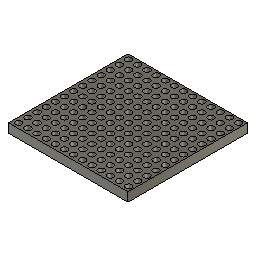
speakergrill_main__unit v1 (Autodesk Fusion 360 design; units mm, degrees)
Autodesk Fusion 360 part; units mm, degrees
sketch "Sketch1" plane through (0, 0, 0) normal (0, 0, 1) x (1, 0, 0)
  line L0 (-122.591, 65.2661) -> (-62.791, 65.2661)
  line L1 (-62.791, 65.2661) -> (-62.791, 5.4661)
  line L2 (-62.791, 5.4661) -> (-122.591, 5.4661)
  line L3 (-122.591, 5.4661) -> (-122.591, 65.2661)
  circle A0 centre (-120, 63) radius 1.5
  circle A1 centre (-115.4167, 63) radius 1.5
  circle A2 centre (-110.8333, 63) radius 1.5
  circle A3 centre (-106.25, 63) radius 1.5
  circle A4 centre (-101.6667, 63) radius 1.5
  circle A5 centre (-97.0833, 63) radius 1.5
  circle A6 centre (-92.5, 63) radius 1.5
  circle A7 centre (-87.9167, 63) radius 1.5
  circle A8 centre (-83.3333, 63) radius 1.5
  circle A9 centre (-78.75, 63) radius 1.5
  circle A10 centre (-74.1667, 63) radius 1.5
  circle A11 centre (-69.5833, 63) radius 1.5
  circle A12 centre (-65, 63) radius 1.5
  circle A13 centre (-120, 58.4167) radius 1.5
  circle A14 centre (-115.4167, 58.4167) radius 1.5
  circle A15 centre (-110.8333, 58.4167) radius 1.5
  circle A16 centre (-106.25, 58.4167) radius 1.5
  circle A17 centre (-101.6667, 58.4167) radius 1.5
  circle A18 centre (-97.0833, 58.4167) radius 1.5
  circle A19 centre (-92.5, 58.4167) radius 1.5
  circle A20 centre (-87.9167, 58.4167) radius 1.5
  circle A21 centre (-83.3333, 58.4167) radius 1.5
  circle A22 centre (-78.75, 58.4167) radius 1.5
  circle A23 centre (-74.1667, 58.4167) radius 1.5
  circle A24 centre (-69.5833, 58.4167) radius 1.5
  circle A25 centre (-65, 58.4167) radius 1.5
  circle A26 centre (-120, 53.8333) radius 1.5
  circle A27 centre (-115.4167, 53.8333) radius 1.5
  circle A28 centre (-110.8333, 53.8333) radius 1.5
  circle A29 centre (-106.25, 53.8333) radius 1.5
  circle A30 centre (-101.6667, 53.8333) radius 1.5
  circle A31 centre (-97.0833, 53.8333) radius 1.5
  circle A32 centre (-92.5, 53.8333) radius 1.5
  circle A33 centre (-87.9167, 53.8333) radius 1.5
  circle A34 centre (-83.3333, 53.8333) radius 1.5
  circle A35 centre (-78.75, 53.8333) radius 1.5
  circle A36 centre (-74.1667, 53.8333) radius 1.5
  circle A37 centre (-69.5833, 53.8333) radius 1.5
  circle A38 centre (-65, 53.8333) radius 1.5
  circle A39 centre (-120, 49.25) radius 1.5
  circle A40 centre (-115.4167, 49.25) radius 1.5
  circle A41 centre (-110.8333, 49.25) radius 1.5
  circle A42 centre (-106.25, 49.25) radius 1.5
  circle A43 centre (-101.6667, 49.25) radius 1.5
  circle A44 centre (-97.0833, 49.25) radius 1.5
  circle A45 centre (-92.5, 49.25) radius 1.5
  circle A46 centre (-87.9167, 49.25) radius 1.5
  circle A47 centre (-83.3333, 49.25) radius 1.5
  circle A48 centre (-78.75, 49.25) radius 1.5
  circle A49 centre (-74.1667, 49.25) radius 1.5
  circle A50 centre (-69.5833, 49.25) radius 1.5
  circle A51 centre (-65, 49.25) radius 1.5
  circle A52 centre (-120, 44.6667) radius 1.5
  circle A53 centre (-115.4167, 44.6667) radius 1.5
  circle A54 centre (-110.8333, 44.6667) radius 1.5
  circle A55 centre (-106.25, 44.6667) radius 1.5
  circle A56 centre (-101.6667, 44.6667) radius 1.5
  circle A57 centre (-97.0833, 44.6667) radius 1.5
  circle A58 centre (-92.5, 44.6667) radius 1.5
  circle A59 centre (-87.9167, 44.6667) radius 1.5
  circle A60 centre (-83.3333, 44.6667) radius 1.5
  circle A61 centre (-78.75, 44.6667) radius 1.5
  circle A62 centre (-74.1667, 44.6667) radius 1.5
  circle A63 centre (-69.5833, 44.6667) radius 1.5
  circle A64 centre (-65, 44.6667) radius 1.5
  circle A65 centre (-120, 40.0833) radius 1.5
  circle A66 centre (-115.4167, 40.0833) radius 1.5
  circle A67 centre (-110.8333, 40.0833) radius 1.5
  circle A68 centre (-106.25, 40.0833) radius 1.5
  circle A69 centre (-101.6667, 40.0833) radius 1.5
  circle A70 centre (-97.0833, 40.0833) radius 1.5
  circle A71 centre (-92.5, 40.0833) radius 1.5
  circle A72 centre (-87.9167, 40.0833) radius 1.5
  circle A73 centre (-83.3333, 40.0833) radius 1.5
  circle A74 centre (-78.75, 40.0833) radius 1.5
  circle A75 centre (-74.1667, 40.0833) radius 1.5
  circle A76 centre (-69.5833, 40.0833) radius 1.5
  circle A77 centre (-65, 40.0833) radius 1.5
  circle A78 centre (-120, 35.5) radius 1.5
  circle A79 centre (-115.4167, 35.5) radius 1.5
  circle A80 centre (-110.8333, 35.5) radius 1.5
  circle A81 centre (-106.25, 35.5) radius 1.5
  circle A82 centre (-101.6667, 35.5) radius 1.5
  circle A83 centre (-97.0833, 35.5) radius 1.5
  circle A84 centre (-92.5, 35.5) radius 1.5
  circle A85 centre (-87.9167, 35.5) radius 1.5
  circle A86 centre (-83.3333, 35.5) radius 1.5
  circle A87 centre (-78.75, 35.5) radius 1.5
  circle A88 centre (-74.1667, 35.5) radius 1.5
  circle A89 centre (-69.5833, 35.5) radius 1.5
  circle A90 centre (-65, 35.5) radius 1.5
  circle A91 centre (-120, 30.9167) radius 1.5
  circle A92 centre (-115.4167, 30.9167) radius 1.5
  circle A93 centre (-110.8333, 30.9167) radius 1.5
  circle A94 centre (-106.25, 30.9167) radius 1.5
  circle A95 centre (-101.6667, 30.9167) radius 1.5
  circle A96 centre (-97.0833, 30.9167) radius 1.5
  circle A97 centre (-92.5, 30.9167) radius 1.5
  circle A98 centre (-87.9167, 30.9167) radius 1.5
  circle A99 centre (-83.3333, 30.9167) radius 1.5
  circle A100 centre (-78.75, 30.9167) radius 1.5
  circle A101 centre (-74.1667, 30.9167) radius 1.5
  circle A102 centre (-69.5833, 30.9167) radius 1.5
  circle A103 centre (-65, 30.9167) radius 1.5
  circle A104 centre (-120, 26.3333) radius 1.5
  circle A105 centre (-115.4167, 26.3333) radius 1.5
  circle A106 centre (-110.8333, 26.3333) radius 1.5
  circle A107 centre (-106.25, 26.3333) radius 1.5
  circle A108 centre (-101.6667, 26.3333) radius 1.5
  circle A109 centre (-97.0833, 26.3333) radius 1.5
  circle A110 centre (-92.5, 26.3333) radius 1.5
  circle A111 centre (-87.9167, 26.3333) radius 1.5
  circle A112 centre (-83.3333, 26.3333) radius 1.5
  circle A113 centre (-78.75, 26.3333) radius 1.5
  circle A114 centre (-74.1667, 26.3333) radius 1.5
  circle A115 centre (-69.5833, 26.3333) radius 1.5
  circle A116 centre (-65, 26.3333) radius 1.5
  circle A117 centre (-120, 21.75) radius 1.5
  circle A118 centre (-115.4167, 21.75) radius 1.5
  circle A119 centre (-110.8333, 21.75) radius 1.5
  circle A120 centre (-106.25, 21.75) radius 1.5
  circle A121 centre (-101.6667, 21.75) radius 1.5
  circle A122 centre (-97.0833, 21.75) radius 1.5
  circle A123 centre (-92.5, 21.75) radius 1.5
  circle A124 centre (-87.9167, 21.75) radius 1.5
  circle A125 centre (-83.3333, 21.75) radius 1.5
  circle A126 centre (-78.75, 21.75) radius 1.5
  circle A127 centre (-74.1667, 21.75) radius 1.5
  circle A128 centre (-69.5833, 21.75) radius 1.5
  circle A129 centre (-65, 21.75) radius 1.5
  circle A130 centre (-120, 17.1667) radius 1.5
  circle A131 centre (-115.4167, 17.1667) radius 1.5
  circle A132 centre (-110.8333, 17.1667) radius 1.5
  circle A133 centre (-106.25, 17.1667) radius 1.5
  circle A134 centre (-101.6667, 17.1667) radius 1.5
  circle A135 centre (-97.0833, 17.1667) radius 1.5
  circle A136 centre (-92.5, 17.1667) radius 1.5
  circle A137 centre (-87.9167, 17.1667) radius 1.5
  circle A138 centre (-83.3333, 17.1667) radius 1.5
  circle A139 centre (-78.75, 17.1667) radius 1.5
  circle A140 centre (-74.1667, 17.1667) radius 1.5
  circle A141 centre (-69.5833, 17.1667) radius 1.5
  circle A142 centre (-65, 17.1667) radius 1.5
  circle A143 centre (-120, 12.5833) radius 1.5
  circle A144 centre (-115.4167, 12.5833) radius 1.5
  circle A145 centre (-110.8333, 12.5833) radius 1.5
  circle A146 centre (-106.25, 12.5833) radius 1.5
  circle A147 centre (-101.6667, 12.5833) radius 1.5
  circle A148 centre (-97.0833, 12.5833) radius 1.5
  circle A149 centre (-92.5, 12.5833) radius 1.5
  circle A150 centre (-87.9167, 12.5833) radius 1.5
  circle A151 centre (-83.3333, 12.5833) radius 1.5
  circle A152 centre (-78.75, 12.5833) radius 1.5
  circle A153 centre (-74.1667, 12.5833) radius 1.5
  circle A154 centre (-69.5833, 12.5833) radius 1.5
  circle A155 centre (-65, 12.5833) radius 1.5
  circle A156 centre (-120, 8) radius 1.5
  circle A157 centre (-115.4167, 8) radius 1.5
  circle A158 centre (-110.8333, 8) radius 1.5
  circle A159 centre (-106.25, 8) radius 1.5
  circle A160 centre (-101.6667, 8) radius 1.5
  circle A161 centre (-97.0833, 8) radius 1.5
  circle A162 centre (-92.5, 8) radius 1.5
  circle A163 centre (-87.9167, 8) radius 1.5
  circle A164 centre (-83.3333, 8) radius 1.5
  circle A165 centre (-78.75, 8) radius 1.5
  circle A166 centre (-74.1667, 8) radius 1.5
  circle A167 centre (-69.5833, 8) radius 1.5
  circle A168 centre (-65, 8) radius 1.5
  dimension "d2" = 59.8
  dimension "d3" = 59.8
  dimension "d4" = 3
  dimension "d7" = 55
  dimension "d8" = -55
  constraint horizontal L0
  constraint vertical L1
  constraint horizontal L2
  constraint vertical L3
  measures "d2" distance of L0.start L0.end
  measures "d3" distance of L0.start L2.end
  measures "d4" diameter of A0
extrude "Extrude1" add sketch "Sketch1" along normal blind 4.5
equation "box_with_depth = 59.80 mm"
equation "d2 = box_with_depth"
equation "d3 = box_with_depth"
